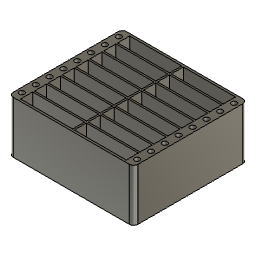
toolbox (Autodesk Fusion 360 design; units mm, degrees)
Autodesk Fusion 360 part; units mm, degrees
sketch "Sketch2" plane through (0, 0, 0) normal (0, 0, 1) x (1, 0, 0)
  line L0 (0, 0) -> (127, 0)
  line L1 (127, 0) -> (127, 131)
  line L2 (127, 131) -> (0, 131)
  line L3 (0, 131) -> (0, 0)
  line L4 (0, 131) -> (127, 0) construction
  line L5 (124.5, 2.5) -> (2.5, 2.5)
  line L6 (2.5, 2.5) -> (2.5, 128.5)
  line L7 (2.5, 128.5) -> (124.5, 128.5)
  line L8 (124.5, 128.5) -> (124.5, 2.5)
  line L9 (124.5, 2.5) -> (2.5, 128.5) construction
  line L10 (2.5, 2.5) -> (124.5, 128.5) construction
  line L11 (63.5, 128.5) -> (63.5, 2.5) construction
  line L12 (64.5, 2.5) -> (62.5, 2.5)
  line L13 (62.5, 2.5) -> (62.5, 128.5)
  line L14 (62.5, 128.5) -> (64.5, 128.5)
  line L15 (64.5, 128.5) -> (64.5, 2.5)
  line L16 (64.5, 2.5) -> (62.5, 128.5) construction
  line L17 (62.5, 2.5) -> (64.5, 128.5) construction
  line L18 (2.5, 128.5) -> (62.5, 128.5)
  line L19 (62.5, 128.5) -> (62.5, 114.5)
  line L20 (62.5, 114.5) -> (2.5, 114.5)
  line L21 (2.5, 114.5) -> (2.5, 128.5)
  line L22 (2.5, 114.5) -> (62.5, 114.5)
  line L23 (62.5, 114.5) -> (62.5, 112.5)
  line L24 (62.5, 112.5) -> (2.5, 112.5)
  line L25 (2.5, 112.5) -> (2.5, 114.5)
  line L26 (62.5, 96.5) -> (2.5, 96.5)
  line L27 (62.5, 98.5) -> (2.5, 98.5)
  line L28 (62.5, 80.5) -> (2.5, 80.5)
  line L29 (62.5, 82.5) -> (2.5, 82.5)
  line L30 (62.5, 64.5) -> (2.5, 64.5)
  line L31 (62.5, 66.5) -> (2.5, 66.5)
  line L32 (62.5, 48.5) -> (2.5, 48.5)
  line L33 (62.5, 50.5) -> (2.5, 50.5)
  line L34 (62.5, 32.5) -> (2.5, 32.5)
  line L35 (62.5, 34.5) -> (2.5, 34.5)
  line L36 (62.5, 16.5) -> (2.5, 16.5)
  line L37 (62.5, 18.5) -> (2.5, 18.5)
  line L38 (124.5, 112.5) -> (64.5, 112.5)
  line L39 (124.5, 114.5) -> (64.5, 114.5)
  line L40 (124.5, 96.5) -> (64.5, 96.5)
  line L41 (124.5, 98.5) -> (64.5, 98.5)
  line L42 (124.5, 80.5) -> (64.5, 80.5)
  line L43 (124.5, 82.5) -> (64.5, 82.5)
  line L44 (124.5, 64.5) -> (64.5, 64.5)
  line L45 (124.5, 66.5) -> (64.5, 66.5)
  line L46 (124.5, 48.5) -> (64.5, 48.5)
  line L47 (124.5, 50.5) -> (64.5, 50.5)
  line L48 (124.5, 32.5) -> (64.5, 32.5)
  line L49 (124.5, 34.5) -> (64.5, 34.5)
  line L50 (124.5, 16.5) -> (64.5, 16.5)
  line L51 (124.5, 18.5) -> (64.5, 18.5)
  line L52 (0, 131) -> (0, 121.5) construction
  line L53 (0, 121.5) -> (-3, 121.5) construction
  circle A0 centre (-3, 121.5) radius 3
  line L54 (0, 131) -> (-8.5, 131) construction
  line L55 (-8.5, 131) -> (135.5, 131)
  line L56 (135.5, 131) -> (135.5, 0)
  line L57 (135.5, 0) -> (-8.5, 0)
  line L58 (-8.5, 0) -> (-8.5, 131)
  line L59 (-8.5, 131) -> (135.5, 0) construction
  line L60 (135.5, 131) -> (-8.5, 0) construction
  circle A1 centre (130, 121.5) radius 3
  circle A2 centre (-3, 105.5) radius 3
  circle A3 centre (130, 105.5) radius 3
  circle A4 centre (-3, 89.5) radius 3
  circle A5 centre (130, 89.5) radius 3
  circle A6 centre (-3, 73.5) radius 3
  circle A7 centre (130, 73.5) radius 3
  circle A8 centre (-3, 57.5) radius 3
  circle A9 centre (130, 57.5) radius 3
  circle A10 centre (-3, 41.5) radius 3
  circle A11 centre (130, 41.5) radius 3
  circle A12 centre (-3, 25.5) radius 3
  circle A13 centre (130, 25.5) radius 3
  circle A14 centre (-3, 9.5) radius 3
  circle A15 centre (130, 9.5) radius 3
  point P0 (63.5, 65.5)
  point P1 (63.5, 65.5)
  point P2 (63.5, 65.5)
  dimension "d44" = 127
  dimension "d45" = 131
  dimension "d46" = 126
  dimension "d47" = 122
  dimension "d48" = 2
  dimension "d49" = 14
  dimension "d50" = 2
  dimension "d53" = 62
  dimension "d61" = 9.5
  dimension "d62" = 3
  dimension "d63" = 6
  dimension "d64" = 8.5
  dimension "d68" = 133
  constraint horizontal L0
  constraint vertical L1
  constraint horizontal L2
  constraint vertical L3
  constraint coincident L0.start L3.end
  constraint horizontal L5
  constraint perpendicular L5 L6
  constraint parallel L5 L7
  constraint parallel L6 L8
  constraint coincident L9 P2
  constraint coincident L10 P2
  constraint midpoint L4 P2
  constraint midpoint L7 L11.start
  constraint midpoint L5 L11.end
  constraint horizontal L12
  constraint perpendicular L12 L13
  constraint parallel L12 L14
  constraint parallel L13 L15
  constraint coincident L5 L12.start
  constraint coincident L16 P2
  constraint coincident L17 P2
  constraint coincident P2 P1
  constraint horizontal L18
  constraint vertical L19
  constraint horizontal L20
  constraint vertical L21
  constraint coincident L13 L19.end
  constraint horizontal L22
  constraint vertical L23
  constraint horizontal L24
  constraint vertical L25
  constraint coincident L13 L23.end
  constraint vertical L52
  constraint horizontal L53
  constraint coincident L53.end A0.centre
  constraint horizontal L54
  constraint horizontal L55
  constraint perpendicular L55 L56
  constraint parallel L55 L57
  constraint parallel L56 L58
  constraint coincident L59 P2
  constraint coincident L60 P2
  measures "d44" distance of L0.start L0.end
  measures "d45" distance of L0.start L2.end
  measures "d46" distance of L5.end L6.end
  measures "d47" distance of L5.start L5.end
  measures "d48" distance of L13.end L14.end
  measures "d49" distance of L6.end L20.end
  measures "d50" distance of L20.end L24.end
  measures "d61" distance of L2.end L52.end
  measures "d62" distance of L52.end L53.end
  measures "d63" diameter of A0
  measures "d64" distance of L2.end L54.end
extrude "Extrude7" add sketch "Sketch2" along normal blind 2.5 contours L0 L1 L2 L3 L55 L57 | A14 | A12 | A10 | A8 | A6 | A4 | A2 | A0 | L3 L55 L57 L58 | A1 | A3 | A5 | A7 | A9 | A11 | A13 | A15 | L1 L55 L56 L57 | L5 L8 L15 L50 | L5 L7 L12 L13 L14 L15 L19 L23 | L8 L15 L50 L51 | L5 L6 L13 L36 | L8 L15 L48 L51 | L6 L13 L36 L37 | L8 L15 L48 L49 | L6 L13 L34 L37 | L8 L15 L46 L49 | L6 L13 L34 L35 | L8 L15 L46 L47 | L6 L13 L32 L35 | L8 L15 L44 L47 | L6 L13 L32 L33 | L8 L15 L44 L45 | L6 L13 L30 L33 | L8 L15 L42 L45 | L6 L13 L30 L31 | L8 L15 L42 L43 | L6 L13 L28 L31 | L8 L15 L40 L43 | L6 L13 L28 L29 | L8 L15 L40 L41 | L6 L13 L26 L29 | L8 L15 L38 L41 | L6 L13 L26 L27 | L8 L15 L38 L39 | L6 L13 L24 L27 | L7 L8 L15 L39 | L6 L13 L20 L22 L23 L24 L25 | L6 L7 L13 L18 L19 L20 L21 L22
extrude "Extrude8" add sketch "Sketch2" along normal blind 60 contours L0 L1 L2 L3 L55 L57 | L3 L55 L57 L58 | L1 L55 L56 L57 | L5 L7 L12 L13 L14 L15 L19 L23 | L8 L15 L50 L51 | L6 L13 L36 L37 | L8 L15 L48 L49 | L6 L13 L34 L35 | L8 L15 L46 L47 | L6 L13 L32 L33 | L8 L15 L44 L45 | L6 L13 L30 L31 | L8 L15 L42 L43 | L6 L13 L28 L29 | L8 L15 L40 L41 | L6 L13 L26 L27 | L8 L15 L38 L39 | L6 L13 L20 L22 L23 L24 L25
fillet "Fillet4" radius 5 4 edges at (135.5, 131, 30) (-8.5, 131, 30) (-8.5, 0, 30) (135.5, 0, 30)
equation "separatorThick = 2 mm"
equation "outerThick = 2.5 mm"
equation "height = 60 mm"
equation "width = 60 mm"
equation "sections = 8"
equation "pocketThick = 14 mm"
equation "d44 = width * 2 + separatorThick + outerThick * 2"
equation "d45 = ( pocketThick + separatorThick ) * sections + outerThick * 2 - separatorThick"
equation "d46 = d45 - outerThick * 2"
equation "d47 = d44 - outerThick * 2"
equation "d48 = separatorThick"
equation "d49 = pocketThick"
equation "d50 = separatorThick"
equation "d52 = sections - 1"
equation "d53 = width + separatorThick"
equation "d54 = -pocketThick - separatorThick"
equation "d61 = pocketThick / 2 + outerThick"
equation "d62 = holesDiam / 2"
equation "d63 = holesDiam"
equation "d64 = holesDiam + outerThick"
equation "holesDiam = 6 mm"
equation "d67 = sections"
equation "d68 = width * 2 + separatorThick + outerThick * 2 + holesDiam"
equation "d69 = -pocketThick - separatorThick"
equation "d70 = outerThick"
equation "d72 = height"
